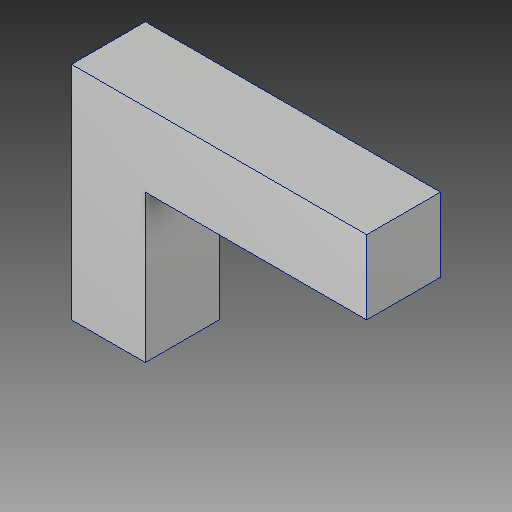
# Autodesk Inventor part: L grab thing
Saved by Autodesk Inventor 2017 (Build 210142000, 142)
## iProperties
Created: 2018-01-31
Part Number: L grab thing
Material: Aluminum 6061
Document SubType Name: Modeling
Designer: S346795925
Density: 2.7 g/cm^3
Appearance: Aluminum - Flat
Author: S346795925
Autodesk Inventor part; units mm, degrees
ref_plane "YZ Plane" through (0, 0, 0) normal (1, 0, 0) x (0, 1, 0)
ref_plane "XZ Plane" through (0, 0, 0) normal (0, 1, 0) x (-1, 0, 0)
ref_plane "XY Plane" through (0, 0, 0) normal (0, 0, 1) x (1, 0, 0)
sketch "Sketch1" plane through (0, 0, 0) normal (0, 0, 1) x (1, 0, 0)
  line L0 (0, 0) -> (0, -76.2)
  line L1 (0, -76.2) -> (25.4, -76.2)
  line L2 (0, 0) -> (101.6, 0)
  line L3 (101.6, 0) -> (101.6, -25.4)
  line L4 (101.6, -25.4) -> (25.4, -25.4)
  line L5 (25.4, -25.4) -> (25.4, -76.2)
  dimension "d0" = 25.4
  dimension "d1" = 25.4
  dimension "d2" = 76.2
  dimension "d5" = 76.2
  constraints: 12 end point, 3 perpendicular, 2 horizontal, 1 vertical
  measures "d0" distance between parallel lines of L4 L2
  measures "d1" distance between parallel lines of L0 L5
  measures "d2" distance between parallel lines of L1 L2
  measures "d5" distance of L3.end L4.end
extrude "Extrusion1" add sketch "Sketch1" along normal blind 25.4
body "Solid1"
